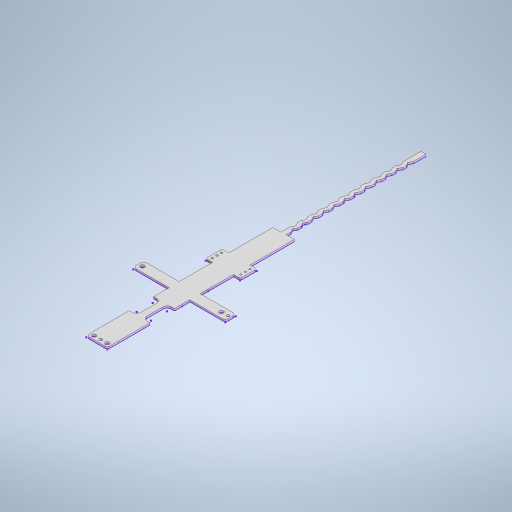
# Autodesk Inventor part: Pinky Finger Part
Saved by Autodesk Inventor 2023.1 (Build 271208000, 208)
## iProperties
Created: 2022-09-21
Part Number: Pinky Finger Part
Material: Generic
Document SubType Name: Modeling
Designer: lxpe222
Density: 1 g/cm^3
Appearance: Default
Author: lxpe222
Autodesk Inventor part; units mm, degrees
ref_plane "YZ Plane" through (0, 0, 0) normal (1, 0, 0) x (0, 1, 0)
ref_plane "XZ Plane" through (0, 0, 0) normal (0, 1, 0) x (-1, 0, 0)
ref_plane "XY Plane" through (0, 0, 0) normal (0, 0, 1) x (1, 0, 0)
sketch "Sketch1" plane through (0, 0, 0) normal (0, 1, 0) x (-1, 0, 0)
  line L0 (-8.8161, 25.9631) -> (-8.8161, 17.4706)
  line L1 (2.7324, -39.7354) -> (2.7324, -15.4975)
  line L2 (-8.811, 39.3303) -> (-8.811, 61.3101)
  line L3 (-7.311, 62.8101) -> (1.089, 62.8101)
  line L4 (2.589, 61.3101) -> (2.589, 39.2875)
  circle A0 centre (0.414, 60.8401) radius 1.175
  circle A1 centre (-6.816, 60.8401) radius 1.175
  line L5 (-8.8161, 25.9631) -> (-7.0943, 25.9631)
  line L6 (-4.8143, 28.2431) -> (-4.8143, 37.0503)
  line L7 (-7.0943, 39.3303) -> (-8.811, 39.3303)
  line L8 (2.589, 39.2875) -> (0.8739, 39.2875)
  line L9 (-1.4061, 37.0075) -> (-1.4061, 28.2431)
  line L10 (0.8739, 25.9631) -> (2.5667, 25.9631)
  arc A2 (0.8739, 39.2875) -> (-1.4061, 37.0075) centre (0.8739, 37.0075) ccw
  arc A3 (-1.4061, 28.2431) -> (0.8739, 25.9631) centre (0.8739, 28.2431) ccw
  arc A4 (-7.0943, 25.9631) -> (-4.8143, 28.2431) centre (-7.0943, 28.2431) ccw
  arc A5 (-4.8143, 37.0503) -> (-7.0943, 39.3303) centre (-7.0943, 37.0503) ccw
  line L11 (2.5667, 17.4706) -> (20.7324, 17.4706)
  line L12 (22.2324, 15.9706) -> (22.2324, 13.2706)
  line L13 (20.7324, 11.7706) -> (2.7324, 11.7706)
  line L14 (-8.8161, 17.4706) -> (-26.8161, 17.4706)
  line L15 (-28.3161, 15.9706) -> (-28.3161, 13.2706)
  line L16 (-26.8161, 11.7706) -> (-8.8161, 11.7706)
  line L17 (2.7324, -6.4975) -> (5.4178, -6.4975)
  line L18 (6.4178, -7.4975) -> (6.4178, -14.4975)
  line L19 (5.4178, -15.4975) -> (2.7324, -15.4975)
  line L20 (-8.8161, -6.4975) -> (-11.5061, -6.4975)
  line L21 (-12.5061, -7.4975) -> (-12.5061, -14.4975)
  line L22 (-11.5061, -15.4975) -> (-8.8161, -15.4975)
  circle A6 centre (-3.2163, 60.7901) radius 0.85
  circle A7 centre (-10.8508, -10.9975) radius 0.5
  circle A8 centre (-10.8508, -13.4975) radius 0.5
  circle A9 centre (4.7625, -10.9975) radius 0.5
  circle A10 centre (4.7625, -13.4975) radius 0.5
  circle A11 centre (-23.3236, 14.6206) radius 1.2
  circle A12 centre (-26.9486, 14.6206) radius 0.825
  circle A13 centre (20.0574, 14.6206) radius 1.2
  line L23 (-8.8161, 11.7706) -> (-8.8161, 3.5293)
  line L24 (2.5667, 17.4706) -> (2.5667, 25.9631)
  line L25 (2.7324, 3.5293) -> (2.7324, 11.7706)
  line L26 (-8.8161, -5.0207) -> (-8.8161, -6.4975)
  line L27 (2.7324, -6.4975) -> (2.7324, -5.0207)
  line L28 (-8.8161, -15.4975) -> (-8.8161, -39.9278)
  arc A14 (2.589, 61.3101) -> (1.089, 62.8101) centre (1.089, 61.3101) ccw
  arc A15 (-7.311, 62.8101) -> (-8.811, 61.3101) centre (-7.311, 61.3101) ccw
  arc A16 (20.7324, 11.7706) -> (22.2324, 13.2706) centre (20.7324, 13.2706) ccw
  arc A17 (22.2324, 15.9706) -> (20.7324, 17.4706) centre (20.7324, 15.9706) ccw
  arc A18 (-28.3161, 13.2706) -> (-26.8161, 11.7706) centre (-26.8161, 13.2706) ccw
  arc A19 (-26.8161, 17.4706) -> (-28.3161, 15.9706) centre (-26.8161, 15.9706) ccw
  line L29 (-8.8161, -39.9278) -> (-4.3275, -39.9278)
  line L30 (-1.734, -39.7356) -> (2.7324, -39.7354)
  line L31 (-1.734, -44.941) -> (-1.734, -39.7356)
  line L32 (-4.3275, -42.4941) -> (-4.3275, -39.9278)
  line L33 (-3.23, -44.3941) -> (-4.3275, -42.4941)
  line L34 (-3.23, -44.3941) -> (-0.6911, -44.3937) construction
  line L35 (-4.2977, -46.2441) -> (-3.23, -44.3941)
  line L36 (-3.2374, -50.1441) -> (-4.2977, -48.2441)
  line L37 (-4.2527, -51.9941) -> (-3.2374, -50.1441)
  line L38 (-3.1764, -55.8941) -> (-4.2527, -53.9941)
  line L39 (-4.2328, -57.7441) -> (-3.1764, -55.8941)
  line L40 (-3.1609, -61.6441) -> (-4.2328, -59.7441)
  line L41 (-4.2364, -63.4941) -> (-3.1609, -61.6441)
  line L42 (-3.1706, -67.3941) -> (-4.2364, -65.4941)
  line L43 (-4.2333, -69.2441) -> (-3.1706, -67.3941)
  line L44 (-3.1482, -73.1435) -> (-4.2333, -71.2441)
  line L45 (-4.3021, -74.9935) -> (-3.1482, -73.1435)
  line L46 (-3.1743, -78.8933) -> (-4.3021, -76.9935)
  line L47 (-4.3415, -80.7433) -> (-3.1743, -78.8933)
  line L48 (-3.2287, -84.7463) -> (-4.3415, -82.7433)
  line L49 (-2.8243, -46.841) -> (-1.7459, -48.691)
  line L50 (-1.734, -44.941) -> (-2.8243, -46.841)
  line L51 (-1.7459, -50.691) -> (-2.7489, -52.591)
  line L52 (-2.7489, -52.591) -> (-1.701, -54.441)
  line L53 (-1.701, -56.441) -> (-2.7244, -58.341)
  line L54 (-2.7244, -58.341) -> (-1.6807, -60.191)
  line L55 (-1.6807, -62.191) -> (-2.7304, -64.091)
  line L56 (-2.7304, -64.091) -> (-1.6926, -65.941)
  line L57 (-1.6926, -67.941) -> (-2.7453, -69.841)
  line L58 (-2.7453, -69.841) -> (-1.6697, -71.691)
  line L59 (-1.6697, -73.691) -> (-2.7357, -75.591)
  line L60 (-2.7357, -75.591) -> (-1.6601, -77.441)
  line L61 (-1.7329, -79.9664) -> (-2.6912, -81.8664)
  line L62 (-2.6912, -81.8664) -> (-1.5867, -83.7164)
  line L63 (-1.7329, -79.9664) -> (-1.6601, -79.441)
  line L64 (-4.3021, -74.9935) -> (-4.3021, -76.9935)
  line L65 (-4.3415, -80.7433) -> (-4.3415, -82.7433)
  line L66 (-4.2364, -63.4941) -> (-4.2364, -65.4941)
  line L67 (-4.2333, -69.2441) -> (-4.2333, -71.2441)
  line L68 (-4.2977, -46.2441) -> (-4.2977, -48.2441)
  line L69 (-4.2527, -51.9941) -> (-4.2527, -53.9941)
  line L70 (-4.2328, -57.7441) -> (-4.2328, -59.7441)
  line L71 (-1.7459, -50.691) -> (-1.7459, -48.691)
  line L72 (-1.701, -56.441) -> (-1.701, -54.441)
  line L73 (-1.6807, -62.191) -> (-1.6807, -60.191)
  line L74 (-1.6926, -67.941) -> (-1.6926, -65.941)
  line L75 (-1.6601, -79.441) -> (-1.6601, -77.441)
  line L76 (-1.6697, -73.691) -> (-1.6697, -71.691)
  line L77 (-3.372, -107.7025) -> (-4.425, -109.6172)
  line L78 (-3.372, -107.7025) -> (-4.425, -105.8672)
  line L79 (-3.2287, -84.7463) -> (-4.3098, -86.6211)
  line L80 (-3.2659, -101.9605) -> (-4.2167, -100.123)
  line L81 (-3.2659, -101.9605) -> (-4.425, -103.8672)
  line L82 (-3.1633, -96.2495) -> (-4.2167, -94.3699)
  line L83 (-3.1633, -96.2495) -> (-4.2167, -98.1199)
  line L84 (-3.2112, -90.502) -> (-4.313, -88.6211)
  line L85 (-3.2112, -90.502) -> (-4.2167, -92.3699)
  line L86 (-2.6377, -93.4434) -> (-1.6273, -95.2161)
  line L87 (-2.6377, -93.4434) -> (-1.5867, -91.4664)
  line L88 (-2.6396, -87.6366) -> (-1.5867, -89.4664)
  line L89 (-2.6396, -87.6366) -> (-1.5867, -85.7164)
  line L90 (-2.7876, -104.8594) -> (-1.7343, -106.7156)
  line L91 (-2.7876, -104.8594) -> (-1.7343, -102.9656)
  line L92 (-2.7339, -99.0686) -> (-1.6273, -97.2172)
  line L93 (-2.7339, -99.0686) -> (-1.7343, -100.9656)
  line L94 (-4.3098, -86.6211) -> (-4.313, -88.6211)
  line L95 (-1.5867, -83.7164) -> (-1.5867, -85.7164)
  line L96 (-1.5867, -89.4664) -> (-1.5867, -91.4664)
  line L97 (-1.6273, -95.2161) -> (-1.6273, -97.2172)
  line L98 (-4.2167, -94.3699) -> (-4.2167, -92.3699)
  line L99 (-4.2167, -98.1199) -> (-4.2167, -100.123)
  line L100 (-1.7343, -100.9656) -> (-1.7343, -102.9656)
  line L101 (-4.425, -103.8672) -> (-4.425, -105.8672)
  line L102 (-1.7343, -106.7156) -> (-1.7343, -116.6072)
  line L103 (-1.7343, -116.6072) -> (-4.425, -116.6072)
  line L104 (-4.425, -116.6072) -> (-4.425, -109.6172)
  line L105 (-8.8161, -5.0207) -> (-8.8161, 3.5293)
  line L106 (2.7324, -5.0207) -> (2.7324, 3.5293)
  circle A20 centre (-10.8508, -8.4975) radius 0.5
  circle A21 centre (4.7625, -8.4975) radius 0.5
  arc A22 (5.4178, -15.4975) -> (6.4178, -14.4975) centre (5.4178, -14.4975) ccw
  arc A23 (6.4178, -7.4975) -> (5.4178, -6.4975) centre (5.4178, -7.4975) ccw
  arc A24 (-11.5061, -6.4975) -> (-12.5061, -7.4975) centre (-11.5061, -7.4975) ccw
  arc A25 (-12.5061, -14.4975) -> (-11.5061, -15.4975) centre (-11.5061, -14.4975) ccw
  point P0 (-8.811, 62.8101)
  point P1 (2.589, 62.8101)
  point P2 (-6.9279, 18.3671)
  point P3 (0.6606, 18.3671)
  point P4 (-6.9323, 25.0551)
  point P5 (22.2324, 11.7706)
  point P6 (22.2324, 17.4706)
  point P7 (-28.3161, 11.7706)
  point P8 (-28.3161, 17.4706)
  point P9 (6.4178, -15.4975)
  point P10 (6.4178, -6.4975)
  point P11 (-12.5061, -15.4975)
  point P12 (-12.5061, -6.4975)
  point P13 (-3.7676, -49.1941)
  point P14 (-3.6908, -72.1938)
  point P15 (-3.7382, -77.9434)
  point P16 (-2.139, -82.7914)
  point P17 (-3.7451, -51.0691)
  point P18 (-8.8161, 21.7168)
  point P19 (-8.8161, 7.6499)
  point P20 (2.7324, 7.6499)
  point P21 (-28.3161, 15.4069)
  point P22 (-28.3161, 13.8342)
  dimension "d275" = 1
  dimension "d276" = 2.4
  dimension "d277" = 2.4
  dimension "d280" = 1.5
  dimension "d281" = 2.35
  dimension "d282" = 2.35
  dimension "d284" = 1.65
  dimension "d286" = 1.7
  dimension "d288" = 0.795
  dimension "d289" = 0.795
  dimension "d290" = 1.17
  dimension "d291" = 1.6
  dimension "d292" = 1.575
  dimension "d293" = 1.5
  dimension "d294" = 1.5
  dimension "d296" = 0.975
  dimension "d297" = 2.175
  dimension "d313" = 9
  dimension "d389" = 120
  dimension "d390" = 120
  dimension "d391" = 2
  dimension "d392" = 2
  dimension "d393" = 2
  dimension "d394" = 2
  dimension "d395" = 2
  dimension "d396" = 2
  dimension "d397" = 2
  dimension "d398" = 2
  dimension "d399" = 2
  dimension "d400" = 2
  dimension "d401" = 2
  dimension "d402" = 2
  dimension "d403" = 2
  dimension "d404" = 2
  dimension "d405" = 2
  dimension "d406" = 2.0032
  dimension "d407" = 2
  dimension "d408" = 2
  dimension "d409" = 3.75
  dimension "d410" = 3.75
  dimension "d411" = 3.75
  dimension "d412" = 3.75
  dimension "d413" = 3.75
  dimension "d414" = 3.75
  dimension "d415" = 3.75
  dimension "d416" = 3.75
  dimension "d417" = 3.75
  dimension "d418" = 3.75
  dimension "d419" = 3.75
  dimension "d420" = 3.75
  dimension "d421" = 3.75
  dimension "d422" = 3.75
  dimension "d423" = 1.85
  dimension "d424" = 1.85
  dimension "d425" = 1.85
  dimension "d426" = 1.85
  dimension "d427" = 1.85
  dimension "d428" = 1.85
  dimension "d429" = 1.85
  dimension "d430" = 1.85
  dimension "d431" = 1.85
  dimension "d432" = 1.85
  dimension "d433" = 1.85
  dimension "d434" = 1.85
  constraints: 215 end point, 69 parallel, 28 point on circle, 28 point on line, 28 tangent, 26 centre point, 11 vertical, 8 equal radius, 8 midpoint, 8 perpendicular, 7 horizontal, 1 collinear
  measures "d275" diameter of A7
  measures "d276" diameter of A11
  measures "d277" diameter of A13
  measures "d280" radius of A14
  measures "d281" diameter of A0
  measures "d282" diameter of A1
  measures "d284" diameter of A12
  measures "d286" diameter of A6
  measures "d288" distance edge to line of A1 L3
  measures "d289" distance edge to line of A0 L3
  measures "d290" distance edge to line of A6 L3
  measures "d293" radius of A16
  measures "d294" radius of A18
  measures "d296" distance edge to line of A13 L12
  measures "d297" distance from line of L4 A0.centre
  measures "d313" distance of point (6.418, -6.497) point (6.418, -15.497)
  measures "d389" angle of L34 L33
  measures "d390" angle of L35 L34
  measures "d391" distance of L71.start L49.end
  measures "d392" distance of L35.start L68.end
  measures "d393" distance of L69.start L38.end
  measures "d394" distance of L53.start L72.end
  measures "d395" distance of L70.start L70.end
  measures "d396" distance of L73.start L54.end
  measures "d397" distance of L66.start L42.end
  measures "d398" distance of L57.start L74.end
  measures "d399" distance of L67.start L44.end
  measures "d400" distance of L76.start L58.end
  measures "d401" distance of L45.start L46.end
  measures "d402" distance of L63.end L75.end
  measures "d403" distance of L47.start L65.end
  measures "d404" distance from line of point (-3.768, -49.194) L49
  measures "d405" distance between parallel lines of L38 L52
  measures "d406" distance between parallel lines of L40 L54
  measures "d407" distance between parallel lines of L42 L56
  measures "d408" distance from line of point (-3.691, -72.194) L58
  measures "d409" vertical distance of L62.end L61.start
  measures "d410" distance of L46.end L47.start
  measures "d411" distance of L75.end L76.start
  measures "d412" vertical distance of L57.start L58.end
  measures "d413" distance of L45.start L44.end
  measures "d414" distance of L42.end L67.start
  measures "d415" distance of L73.start L74.end
  measures "d416" distance of L70.end L66.start
  measures "d417" vertical distance of L38.end L70.start
  measures "d418" vertical distance of L53.start L54.end
  measures "d419" vertical distance of L71.start L72.end
  measures "d420" vertical distance of L68.end L69.start
  measures "d421" distance of L31.start L49.end
  measures "d422" vertical distance of L32.start L35.start
  measures "d423" vertical distance of L35.start L34.start
  measures "d424" vertical distance of L69.start L36.start
  measures "d425" vertical distance of L50.end L49.end
  measures "d426" vertical distance of L52.start L72.end
  measures "d427" vertical distance of L70.start L39.end
  measures "d428" vertical distance of L54.end L53.end
  measures "d429" vertical distance of L66.start L40.start
  measures "d430" vertical distance of L56.start L74.end
  measures "d431" vertical distance of L43.end L67.start
  measures "d432" vertical distance of L57.end L58.end
  measures "d433" vertical distance of L59.end L75.end
  measures "d434" vertical distance of L44.start L45.start
extrude "Extrusion8" add sketch "Sketch1" along normal blind 1
body "Solid3"
